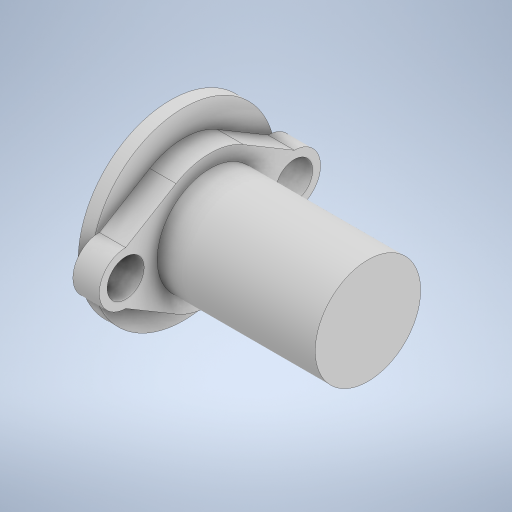
# Autodesk Inventor part: Двигатель ущербный
Saved by Autodesk Inventor 2023 (Build 270158000, 158)
## iProperties
Created: 2022-05-13
Part Number: Двигатель ущербный
Material: Типовые
Document SubType Name: Modeling
Designer: avkap
Density: 1 g/cm^3
Appearance: По умолчанию
Author: avkap
Autodesk Inventor part; units mm, degrees
ref_plane "YZ Plane" through (0, 0, 0) normal (1, 0, 0) x (0, 1, 0)
ref_plane "XZ Plane" through (0, 0, 0) normal (0, 1, 0) x (-1, 0, 0)
ref_plane "XY Plane" through (0, 0, 0) normal (0, 0, 1) x (1, 0, 0)
sketch "Эскиз1" plane through (0, 0, 0) normal (1, 0, 0) x (0, 1, 0)
  circle A0 centre (0, 0) radius 25
  line L0 (0, -25) -> (0, -32)
  line L1 (0, 25) -> (0, 32)
  circle A1 centre (0, 32) radius 7
  circle A2 centre (0, 32) radius 10
  circle A3 centre (0, -32) radius 7
  circle A4 centre (0, -32) radius 10
  line L2 (9.9998, -32.0687) -> (21.4797, -12.7916)
  line L3 (-10, -32) -> (-21.4596, -12.8251)
  line L4 (-10, 32) -> (-20.7737, 13.9088)
  line L5 (10, 32) -> (21.4596, 12.8251)
  dimension "d0" = 50
  dimension "d1" = 7
  dimension "d2" = 7
  dimension "d3" = 20
  dimension "d4" = 20
  constraints: 12 end point, 10 point on circle, 5 coincident, 3 centre point, 3 tangent, 2 point on line, 2 vertical alignment, 1 parallel, 1 vertical, 4 other
  measures "d0" diameter of A0
  measures "d1" distance of L0.start L0.end
  measures "d2" distance of L1.start L1.end
  measures "d3" diameter of A2
  measures "d4" diameter of A4
extrude "Выдавливание1" add sketch "Эскиз1" along normal blind 10
sketch "Эскиз2" plane through (10, 0, 0) normal (1, 0, 0) x (0, 0, -1)
  circle A0 centre (0, 0) radius 20
  dimension "d7" = 40
  constraints: 1 centre point, 1 coincident
  measures "d7" diameter of A0
extrude "Выдавливание2" add sketch "Эскиз2" along normal blind 60
sketch "Эскиз3" plane through (0, 0, 0) normal (-1, 0, 0) x (0, 0, 1)
  circle A0 centre (0, 0) radius 35
  dimension "d10" = 70
  constraints: 1 centre point, 1 coincident
  measures "d10" diameter of A0
extrude "Выдавливание3" add sketch "Эскиз3" along normal blind 5
sketch "Эскиз4" plane through (-5, 0, 0) normal (-1, 0, 0) x (0, 0, 1)
  circle A0 centre (0, 0) radius 16
  circle A1 centre (0, 0) radius 3
  dimension "d13" = 32
  dimension "d16" = 6
  constraints: 2 centre point, 2 coincident
  measures "d13" diameter of A0
  measures "d16" diameter of A1
extrude "Выдавливание4" add sketch "Эскиз4" along normal blind 10
